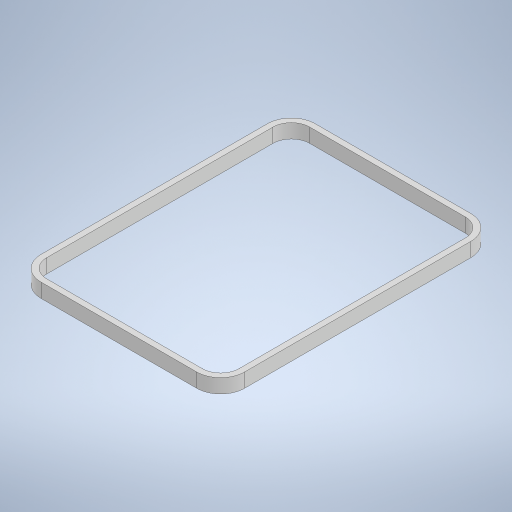
# Autodesk Inventor part: Stand Brace
Saved by Autodesk Inventor 2024.1 (Build 281209000, 209)
## iProperties
Created: 2024-01-03
Part Number: Stand Brace
Material: Generic
Document SubType Name: Modeling
Designer: ryanm
Density: 1 g/cm^3
Appearance: Default
Author: ryanm
Autodesk Inventor part; units mm, degrees
ref_plane "YZ Plane" through (0, 0, 0) normal (1, 0, 0) x (0, 1, 0)
ref_plane "XZ Plane" through (0, 0, 0) normal (0, 1, 0) x (-1, 0, 0)
ref_plane "XY Plane" through (0, 0, 0) normal (0, 0, 1) x (1, 0, 0)
sketch "Sketch1" plane through (0, 0, 0) normal (0, 1, 0) x (-1, 0, 0)
  arc A0 (27.5, -46.5) -> (34, -40) centre (27.5, -40) ccw
  line L0 (36, -40) -> (36, 0)
  line L1 (34, -40) -> (34, 0)
  arc A1 (27.5, -48.5) -> (36, -40) centre (27.5, -40) ccw
  line L2 (27.5, -48.5) -> (0, -48.5)
  line L3 (27.5, -46.5) -> (0, -46.5)
  line L4 (0, -48.5) -> (0, 0) construction
  arc A2 (-34, -40) -> (-27.5, -46.5) centre (-27.5, -40) ccw
  line L5 (-36, -40) -> (-36, 0)
  line L6 (-34, -40) -> (-34, 0)
  arc A3 (-36, -40) -> (-27.5, -48.5) centre (-27.5, -40) ccw
  line L7 (-27.5, -48.5) -> (0, -48.5)
  line L8 (-27.5, -46.5) -> (0, -46.5)
  line L9 (36, 0) -> (-36, 0) construction
  arc A4 (34, 40) -> (27.5, 46.5) centre (27.5, 40) ccw
  line L10 (36, 40) -> (36, 0)
  line L11 (34, 40) -> (34, 0)
  arc A5 (36, 40) -> (27.5, 48.5) centre (27.5, 40) ccw
  line L12 (27.5, 48.5) -> (0, 48.5)
  line L13 (27.5, 46.5) -> (0, 46.5)
  line L14 (-27.5, 48.5) -> (0, 48.5)
  arc A6 (-27.5, 46.5) -> (-34, 40) centre (-27.5, 40) ccw
  line L15 (-36, 40) -> (-36, 0)
  line L16 (-34, 40) -> (-34, 0)
  arc A7 (-27.5, 48.5) -> (-36, 40) centre (-27.5, 40) ccw
  line L17 (-27.5, 46.5) -> (0, 46.5)
  dimension "d0" = 13
  dimension "d20" = 2
  dimension "d21" = 2
  dimension "d26" = 40
  dimension "d27" = 27.5
  dimension "d28" = 2
  constraints: 36 end point, 20 symmetric about line, 16 point on circle, 8 centre point, 4 horizontal alignment, 3 horizontal, 3 vertical, 2 tangent, 2 vertical alignment, 1 coincident, 6 other
  measures "d0" diameter of A0
  measures "d20" radial gap between concentric circles of A0 A1
  measures "d21" distance between parallel lines of L0 L1
  measures "d26" distance of L0.start L0.end
  measures "d27" distance of L2.start L2.end
  measures "d28" distance between parallel lines of L3 L2
extrude "Extrusion1" add sketch "Sketch1" along normal blind 5
sketch "Sketch2" plane through (0, 0, 0) normal (0, -1, 0) x (1, 0, 0)
  arc A0 (-34, -40) -> (-27.5, -46.5) centre (-27.5, -40) ccw projected
  arc A1 (-36, -40) -> (-27.5, -48.5) centre (-27.5, -40) ccw projected
  line L0 (-17.5, -46.5) -> (-17.5, -48.5)
  line L1 (17.5, -46.5) -> (17.5, -48.5)
  line L2 (-36, -40) -> (-36, 40) projected
  line L3 (27.5, -48.5) -> (-27.5, -48.5) projected
  arc A2 (27.5, -48.5) -> (36, -40) centre (27.5, -40) ccw projected
  line L4 (36, 40) -> (36, -40) projected
  arc A3 (36, 40) -> (27.5, 48.5) centre (27.5, 40) ccw projected
  line L5 (-27.5, 48.5) -> (27.5, 48.5) projected
  arc A4 (-27.5, 48.5) -> (-36, 40) centre (-27.5, 40) ccw projected
  line L6 (34, -40) -> (34, 40) projected
  arc A5 (27.5, -46.5) -> (34, -40) centre (27.5, -40) ccw projected
  line L7 (-27.5, -46.5) -> (27.5, -46.5) projected
  line L8 (-34, 40) -> (-34, -40) projected
  arc A6 (-27.5, 46.5) -> (-34, 40) centre (-27.5, 40) ccw projected
  line L9 (27.5, 46.5) -> (-27.5, 46.5) projected
  arc A7 (34, 40) -> (27.5, 46.5) centre (27.5, 40) ccw projected
  point P0 (0, 0)
  dimension "d16" = 35
  dimension "d17" = 10
  constraints: 4 end point
  measures "d16" distance between parallel lines of L1 L0
  measures "d17" distance from line of L0 L3.end
extrude "Extrusion2" [suppressed]
equation "\"d21\" = d20"
body "Solid1"
